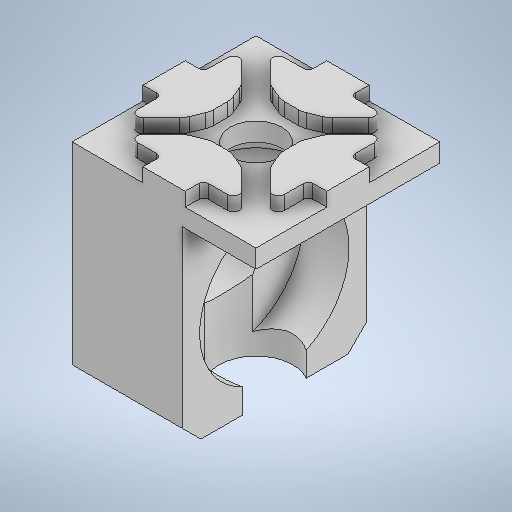
# Autodesk Inventor part: Kondensatorbox
Saved by Autodesk Inventor 2025 (Build 290162010, 162A)
## iProperties
Created: 2024-10-11
Part Number: Kondensatorbox
Material: Generisch
Document SubType Name: Modeling
Designer: max-h
Density: 1 g/cm^3
Appearance: Vorgabe
Author: max-h
Autodesk Inventor part; units mm, degrees
ref_plane "YZ Plane" through (0, 0, 0) normal (1, 0, 0) x (0, 1, 0)
ref_plane "XZ Plane" through (0, 0, 0) normal (0, 1, 0) x (-1, 0, 0)
ref_plane "XY Plane" through (0, 0, 0) normal (0, 0, 1) x (1, 0, 0)
sketch "Skizze10" plane through (0, 0, 0) normal (0, 1, 0) x (-1, 0, 0)
  line L0 (10, 10) -> (-10, 10)
  line L1 (-10, 10) -> (-10, -10)
  line L2 (-10, -10) -> (10, -10)
  line L3 (10, -10) -> (10, 10)
  circle A0 centre (0, 0) radius 2.8
  line L4 (14, 0) -> (-14, 0) projected
  line L5 (0, -14) -> (0, 14) projected
  dimension "d78" = 20
  dimension "d79" = 20
  dimension "d80" = 5.6
  constraints: 8 end point, 2 parallel, 1 centre point, 1 coincident, 1 horizontal, 1 perpendicular, 2 other
  measures "d78" distance of L2.end L0.start
  measures "d79" distance of L0.start L0.end
  measures "d80" diameter of A0
extrude "Extrusion10" add sketch "Skizze10" along normal blind 2 contours L3 L4 A0 L5 L0 | L5 A0 L4 L1 L0 | L3 L2 L5 A0 L4 | L4 A0 L5 L2 L1
sketch "Skizze11" plane through (0, 2, 0) normal (0, 1, 0) x (1, 0, 0)
  line L0 (-2.3, -10) -> (2.3, -10)
  line L1 (-14, 0) -> (14, 0) projected
  line L2 (0, 14) -> (0, -14) projected
  line L3 (-10, -10) -> (10, -10) projected
  line L4 (2.3, -10) -> (2.3, -8.5)
  line L5 (-2.3, -10) -> (-2.3, -8.5)
  arc A0 (2.3, -8.5) -> (2.8, -8) centre (2.8, -8.5) ccw construction
  line L6 (2.8, -8) -> (4.918, -8)
  arc A1 (2.8, -8) -> (2.3, -8.5) centre (2.8, -8.5) ccw
  arc A2 (-2.8, -8) -> (-2.3, -8.5) centre (-2.8, -8.5) ccw construction
  line L7 (-2.8, -8) -> (-4.918, -8)
  arc A3 (-2.3, -8.5) -> (-2.8, -8) centre (-2.8, -8.5) ccw
  arc A4 (5.3649, -6.9211) -> (4.918, -8) centre (4.918, -7.368) ccw construction
  arc A5 (-4.918, -8) -> (-5.3649, -6.9211) centre (-4.918, -7.368) ccw construction
  line L8 (3.1149, -4.6711) -> (5.3649, -6.9211)
  line L9 (-5.3649, -6.9211) -> (-3.1149, -4.6711)
  line L10 (-1.1345, -3.85) -> (1.1345, -3.85)
  line L11 (-3.1149, -4.6711) -> (-1.1345, -3.85)
  line L12 (1.1345, -3.85) -> (3.1149, -4.6711)
  arc A6 (4.918, -8) -> (5.3649, -6.9211) centre (4.918, -7.368) ccw
  arc A7 (-5.3649, -6.9211) -> (-4.918, -8) centre (-4.918, -7.368) ccw
  line L13 (2.3, 10) -> (-2.3, 10)
  line L14 (10, 10) -> (-10, 10) construction
  line L15 (-2.3, 10) -> (-2.3, 8.5)
  line L16 (2.3, 10) -> (2.3, 8.5)
  arc A8 (-2.3, 8.5) -> (-2.8, 8) centre (-2.8, 8.5) ccw construction
  line L17 (-2.8, 8) -> (-4.918, 8)
  arc A9 (-2.8, 8) -> (-2.3, 8.5) centre (-2.8, 8.5) ccw
  arc A10 (2.8, 8) -> (2.3, 8.5) centre (2.8, 8.5) ccw construction
  line L18 (2.8, 8) -> (4.918, 8)
  arc A11 (2.3, 8.5) -> (2.8, 8) centre (2.8, 8.5) ccw
  arc A12 (-5.3649, 6.9211) -> (-4.918, 8) centre (-4.918, 7.368) ccw construction
  arc A13 (4.918, 8) -> (5.3649, 6.9211) centre (4.918, 7.368) ccw construction
  line L19 (-3.1149, 4.6711) -> (-5.3649, 6.9211)
  line L20 (5.3649, 6.9211) -> (3.1149, 4.6711)
  line L21 (1.1345, 3.85) -> (-1.1345, 3.85)
  line L22 (3.1149, 4.6711) -> (1.1345, 3.85)
  line L23 (-1.1345, 3.85) -> (-3.1149, 4.6711)
  arc A14 (-4.918, 8) -> (-5.3649, 6.9211) centre (-4.918, 7.368) ccw
  arc A15 (5.3649, 6.9211) -> (4.918, 8) centre (4.918, 7.368) ccw
  line L24 (10, 10) -> (-10, 10) projected
  line L25 (-10, 2.3) -> (-10, -2.3)
  line L26 (-10, 10) -> (-10, -10) construction
  line L27 (-10, -2.3) -> (-8.5, -2.3)
  line L28 (-10, 2.3) -> (-8.5, 2.3)
  arc A16 (-8.5, -2.3) -> (-8, -2.8) centre (-8.5, -2.8) ccw construction
  line L29 (-8, -2.8) -> (-8, -4.918)
  arc A17 (-8, -2.8) -> (-8.5, -2.3) centre (-8.5, -2.8) ccw
  arc A18 (-8, 2.8) -> (-8.5, 2.3) centre (-8.5, 2.8) ccw construction
  line L30 (-8, 2.8) -> (-8, 4.918)
  arc A19 (-8.5, 2.3) -> (-8, 2.8) centre (-8.5, 2.8) ccw
  arc A20 (-6.9211, -5.3649) -> (-8, -4.918) centre (-7.368, -4.918) ccw construction
  arc A21 (-8, 4.918) -> (-6.9211, 5.3649) centre (-7.368, 4.918) ccw construction
  line L31 (-4.6711, -3.1149) -> (-6.9211, -5.3649)
  line L32 (-6.9211, 5.3649) -> (-4.6711, 3.1149)
  line L33 (-3.85, 1.1345) -> (-3.85, -1.1345)
  line L34 (-4.6711, 3.1149) -> (-3.85, 1.1345)
  line L35 (-3.85, -1.1345) -> (-4.6711, -3.1149)
  arc A22 (-8, -4.918) -> (-6.9211, -5.3649) centre (-7.368, -4.918) ccw
  arc A23 (-6.9211, 5.3649) -> (-8, 4.918) centre (-7.368, 4.918) ccw
  line L36 (3.85, 1.1345) -> (4.6711, 3.1149)
  line L37 (3.85, -1.1345) -> (3.85, 1.1345)
  line L38 (8, 2.8) -> (8, 4.918)
  arc A24 (6.9211, 5.3649) -> (8, 4.918) centre (7.368, 4.918) ccw construction
  arc A25 (8, 2.8) -> (8.5, 2.3) centre (8.5, 2.8) ccw
  arc A26 (8, 4.918) -> (6.9211, 5.3649) centre (7.368, 4.918) ccw
  arc A27 (8.5, 2.3) -> (8, 2.8) centre (8.5, 2.8) ccw construction
  line L39 (10, 2.3) -> (8.5, 2.3)
  line L40 (10, -10) -> (10, 10) construction
  line L41 (10, -2.3) -> (10, 2.3)
  line L42 (4.6711, -3.1149) -> (3.85, -1.1345)
  line L43 (10, -2.3) -> (8.5, -2.3)
  arc A28 (8.5, -2.3) -> (8, -2.8) centre (8.5, -2.8) ccw
  arc A29 (8, -2.8) -> (8.5, -2.3) centre (8.5, -2.8) ccw construction
  line L44 (6.9211, -5.3649) -> (4.6711, -3.1149)
  line L45 (8, -2.8) -> (8, -4.918)
  arc A30 (8, -4.918) -> (6.9211, -5.3649) centre (7.368, -4.918) ccw construction
  arc A31 (6.9211, -5.3649) -> (8, -4.918) centre (7.368, -4.918) ccw
  line L46 (4.6711, 3.1149) -> (6.9211, 5.3649)
  line L47 (10, -10) -> (10, 10) construction
  line L48 (-10, 10) -> (-10, -10) projected
  line L49 (10, -10) -> (10, 10) projected
  line L50 (-8.5, 2.8) -> (-10, 2.8) construction
  line L51 (-8.5, -2.8) -> (-10, -2.8) construction
  line L52 (-2.8, 8.5) -> (-2.8, 10) construction
  line L53 (2.8, 8.5) -> (2.8, 10) construction
  line L54 (8.5, 2.8) -> (10, 2.8) construction
  line L55 (8.5, -2.8) -> (10, -2.8) construction
  line L56 (2.8, -8.5) -> (2.8, -10) construction
  line L57 (-2.8, -8.5) -> (-2.8, -10) construction
  point P0 (0, 0)
  point P1 (4.2399, -5.7961)
  point P2 (-4.2399, 5.7961)
  point P3 (-5.7961, -4.2399)
  point P4 (5.7961, 4.2399)
  dimension "d83" = 4.6
  dimension "d85" = 1
  dimension "d87" = 1.264
  dimension "d89" = 45
  dimension "d90" = 2.118
  dimension "d91" = 45
  dimension "d92" = 3.182
  dimension "d93" = 2.269
  dimension "d94" = 6.15
  dimension "d98" = 4.6
  dimension "d102" = 45
  dimension "d104" = 45
  dimension "d107" = 6.15
  dimension "d108" = 4.6
  dimension "d112" = 45
  dimension "d114" = 45
  dimension "d117" = 6.15
  dimension "d118" = 4.6
  dimension "d119" = 1
  dimension "d122" = 45
  dimension "d124" = 45
  dimension "d127" = 6.15
  dimension "d128" = 1.5
  constraints: 104 end point, 64 point on circle, 32 centre point, 32 tangent, 23 equal length, 13 equal radius, 8 collinear, 8 point on line, 7 perpendicular, 5 symmetric about line, 4 coincident, 4 horizontal, 4 midpoint, 3 parallel, 2 vertical, 6 other
  measures "d83" distance of L0.start L0.end
  measures "d85" diameter of A0
  measures "d87" diameter of A4
  measures "d89" angle of L8 L6
  measures "d90" distance of L6.start L6.end
  measures "d91" angle of L7 L9
  measures "d92" distance of L8.start L8.end
  measures "d93" distance of L10.start L10.end
  measures "d94" distance between parallel lines of L0 L10
  measures "d98" distance of L13.start L15.start
  measures "d102" angle of L19 L17
  measures "d104" angle of L18 L20
  measures "d107" distance between parallel lines of L13 L21
  measures "d108" distance of L25.start L25.end
  measures "d112" angle of L31 L29
  measures "d114" angle of L30 L32
  measures "d117" distance between parallel lines of L25 L33
  measures "d118" distance of L41.start L41.end
  measures "d119" diameter of A27
  measures "d122" angle of L46 L38
  measures "d124" angle of L45 L44
  measures "d127" distance between parallel lines of L41 L37
  measures "d128" distance from line of L26 L50.start
extrude "Extrusion11" add sketch "Skizze11" along normal blind 1.5 contours L5 A3 L7 A7 L9 L11 L10 L2 L0 | L2 L10 L12 L8 A6 L6 A1 L4 L0 | L25 L1 L33 L35 L31 A22 L29 A17 L27 | L25 L28 A19 L30 A23 L32 L34 L33 L1 | L43 A28 L45 A31 L44 L42 L37 L1 L41 | L37 L36 L46 A26 L38 A25 L39 L41 L1 | L21 L23 L19 A14 L17 A9 L15 L13 L2 | L2 L13 L16 A11 L18 A15 L20 L22 L21
fillet "Rundung3" radius 2 16 edges at (3.1149, 2.75, 4.6711) (1.1345, 2.75, 3.85) (-1.1345, 2.75, 3.85) (-3.1149, 2.75, 4.6711) (-3.1149, 2.75, -4.6711) (-1.1345, 2.75, -3.85) (1.1345, 2.75, -3.85) (3.1149, 2.75, -4.6711) (-4.6711, 2.75, 3.1149) (-3.85, 2.75, 1.1345) (-3.85, 2.75, -1.1345) (-4.6711, 2.75, -3.1149) (4.6711, 2.75, 3.1149) (3.85, 2.75, 1.1345) (3.85, 2.75, -1.1345) (4.6711, 2.75, -3.1149)
sketch "Skizze12" plane through (0, 0, 0) normal (0, -1, 0) x (1, 0, 0)
  line L0 (-2.3, -10) -> (-10, -10) projected
  line L1 (-10, 10) -> (2, 10)
  line L2 (2, 10) -> (2, -10)
  line L3 (2, -10) -> (-10, -10)
  line L4 (-10, -10) -> (-10, 10)
  point P0 (0, 0)
  dimension "d129" = 12
  constraints: 8 end point, 2 parallel, 1 horizontal, 1 perpendicular, 1 point on line
  measures "d129" distance between parallel lines of L4 L2
extrude "Extrusion12" add sketch "Skizze12" along normal blind 21
sketch "Skizze16" plane through (0, -21, 0) normal (0, -1, 0) x (1, 0, 0)
  circle A0 centre (0, 0) radius 4
  dimension "d141" = 8
  constraints: 1 centre point, 1 coincident
  measures "d141" diameter of A0
extrude "Extrusion15" cut sketch "Skizze16" against normal blind 21
sketch "Skizze19" plane through (2, 0, 10) normal (1, 0, 0) x (0, 0, -1)
  circle A0 centre (10, -11) radius 3.5
  line L0 (0, 0) -> (0, -21) projected
  line L1 (20, -21) -> (0, -21) projected
  point P0 (10, 0)
  dimension "d147" = 7
  dimension "d148" = 10
  dimension "d149" = 10
  constraints: 1 centre point
  measures "d147" diameter of A0
  measures "d148" distance from line of L0 A0.centre
  measures "d149" distance from line of L1 A0.centre
extrude "Extrusion17" cut sketch "Skizze19" against normal through all
sketch "Skizze20" plane through (2, -21, -10) normal (1, 0, 0) x (0, 0, -1)
  circle A0 centre (-10, 10) radius 3.5 projected
  circle A1 centre (-10, 10) radius 8.125
  point P0 (-10, 21)
  dimension "d152" = 16.25
  constraints: 1 centre point, 1 coincident
  measures "d152" diameter of A1
extrude "Extrusion18" cut sketch "Skizze20" against normal blind 5
chamfer "Fasen4" distance 2 angle 45 2 edges at (-4, -21, -10) (-4, -21, 10)
sketch "Skizze21" plane through (0, 0, 0) normal (0, -1, 0) x (1, 0, 0)
  circle A0 centre (0, 0) radius 4.625
  dimension "d158" = 9.25
  constraints: 1 centre point, 1 coincident
  measures "d158" diameter of A0
extrude "Extrusion19" cut sketch "Skizze21" along normal blind 8
chamfer "Fasen5" distance 1.821 angle 45 1 edges at (-4.625, 0, 0)
chamfer "Fasen6" distance 0.25 angle 45 2 edges at (-3.7298, -8, 2.7349) (-3.7298, -8, -2.7349)
